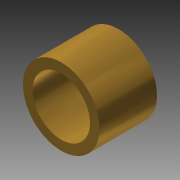
# Autodesk Inventor part: E3DBowdenInsert
Saved by Autodesk Inventor 2015 SP1 (Build 190203100, 203)
## iProperties
Created: 2014-11-28
Part Number: E3DBowdenInsert
Material: Brass, Soft Yellow
Document SubType Name: Modeling
Designer: Jack
Density: 8.47 g/cm^3
Appearance: Brass - Satin
Mass: 1.09652 g
Surface Area: 3.0268 cm^2
Volume: 0.12946 cm^3
Author: Jack
Autodesk Inventor part; units mm, degrees
ref_plane "YZ Plane" through (0, 0, 0) normal (1, 0, 0) x (0, 1, 0)
ref_plane "XZ Plane" through (0, 0, 0) normal (0, 1, 0) x (-1, 0, 0)
ref_plane "XY Plane" through (0, 0, 0) normal (0, 0, 1) x (1, 0, 0)
sketch "Sketch1" plane through (0, 0, 0) normal (0, 1, 0) x (-1, 0, 0)
  circle A0 centre (0, 0) radius 4
  dimension "d0" = 8
  constraints: 1 centre point, 1 coincident
  measures "d0" diameter of A0
extrude "Extrusion1" add sketch "Sketch1" along normal blind 6
sketch "Sketch2" plane through (0, 6, 0) normal (0, 1, 0) x (1, 0, 0)
  circle A0 centre (0, 0) radius 4 projected
  circle A1 centre (0, 0) radius 3
  dimension "d3" = 6
  constraints: 1 centre point, 1 coincident
  measures "d3" diameter of A1
extrude "Extrusion2" cut sketch "Sketch2" against normal up to next contours A1
chamfer "Chamfer1" distance 0.5 angle 45 1 edges at (-3, 6, 0)
body "Solid1"
